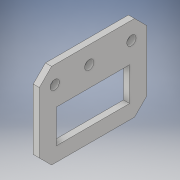
# Autodesk Inventor part: PowerSwitch
Saved by Autodesk Inventor 2017 (Build 210142000, 142)
## iProperties
Created: 2017-10-31
Part Number: PowerSwitch
Material: Generic
Document SubType Name: Modeling
Designer: User
Density: 1 g/cm^3
Appearance: Default
Author: User
Autodesk Inventor part; units mm, degrees
ref_plane "YZ Plane" through (0, 0, 0) normal (1, 0, 0) x (0, 1, 0)
ref_plane "XZ Plane" through (0, 0, 0) normal (0, 1, 0) x (-1, 0, 0)
ref_plane "XY Plane" through (0, 0, 0) normal (0, 0, 1) x (1, 0, 0)
sketch "Sketch1" plane through (0, 0, 0) normal (1, 0, 0) x (0, 1, 0)
  line L0 (0, 0) -> (35.56, 0)
  line L1 (35.56, 0) -> (35.56, -44.704)
  line L2 (35.56, -44.704) -> (0, -44.704)
  line L3 (0, -44.704) -> (0, 0)
  circle A0 centre (28.2956, -38.3286) radius 1.9304
  circle A1 centre (28.2956, -6.3754) radius 1.9304
  circle A2 centre (28.2956, -20.762) radius 1.9304
  line L4 (19.9136, -7.112) -> (5.9436, -7.112)
  line L5 (5.9436, -7.112) -> (5.9436, -37.592)
  line L6 (5.9436, -37.592) -> (19.9136, -37.592)
  line L7 (19.9136, -37.592) -> (19.9136, -7.112)
  dimension "d0" = 35.56
  dimension "d1" = 44.704
  dimension "d2" = 3.8608
  dimension "d3" = 3.8608
  dimension "d4" = 3.8608
  dimension "d5" = 6.3754
  dimension "d6" = 6.3754
  dimension "d7" = 7.2644
  dimension "d8" = 7.2644
  dimension "d9" = 7.2644
  dimension "d10" = 13.97
  dimension "d11" = 30.48
  dimension "d12" = 15.6464
  dimension "d13" = 7.112
  constraints: 16 end point, 4 parallel, 3 centre point, 2 horizontal, 2 perpendicular
  measures "d0" distance of L1.end L2.end
  measures "d1" distance of L0.end L1.end
  measures "d2" diameter of A0
  measures "d3" diameter of A1
  measures "d4" diameter of A2
  measures "d5" distance from line of L2 A0.centre
  measures "d6" distance from line of L0 A1.centre
  measures "d7" distance from line of L1 A0.centre
  measures "d8" distance from line of L1 A1.centre
  measures "d9" distance from line of L1 A2.centre
  measures "d10" distance of L6.end L5.end
  measures "d11" distance of L5.end L4.end
  measures "d12" distance between parallel lines of L1 L7
  measures "d13" distance between parallel lines of L2 L6
extrude "Extrusion1" add sketch "Sketch1" along normal blind 2.54
chamfer "Chamfer1" distance 5.08 angle 45 4 edges at (1.27, 35.56, 0) (1.27, 0, 0) (1.27, 35.56, -44.704) (1.27, 0, -44.704)
equation "\"d6\" = d5"
equation "\"d8\" = d7"
equation "\"d9\" = d7"
equation "\"d13\" = -0.5 * d11 + 0.5 * d1"
body "Solid1"
